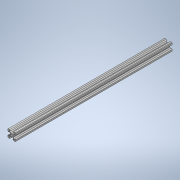
# Autodesk Inventor part: 2020
Saved by Autodesk Inventor 2020 (Build 240168000, 168)
## iProperties
Created: 2021-03-19
Part Number: 2020
Material: Aluminum 6061
Document SubType Name: Modeling
Designer: AOB
Mass: 180.098 g
Surface Area: 658.384 cm^2
Volume: 66.7031 cm^3
Density: 2.7 g/cm^3
Appearance: Anodized - Light Gray
Author: AOB
Autodesk Inventor part; units mm, degrees
ref_plane "YZ Plane" through (0, 0, 0) normal (1, 0, 0) x (0, 1, 0)
ref_plane "XZ Plane" through (0, 0, 0) normal (0, 1, 0) x (-1, 0, 0)
ref_plane "XY Plane" through (0, 0, 0) normal (0, 0, 1) x (1, 0, 0)
sketch "Sketch1" plane through (0, 0, 0) normal (0, 0, 1) x (1, 0, 0)
  line L0 (1, 7) -> (1, 7)
  line L1 (-1, 5) -> (-1, 1)
  arc A0 (-1, 1) -> (0, 0) centre (0, 1) ccw
  line L2 (0, 0) -> (4, 0)
  line L3 (6, 2) -> (6, 2)
  line L4 (6, 2) -> (3, 2)
  line L5 (3, 2) -> (3, 2.9393)
  line L6 (3, 2.9393) -> (6.0607, 6)
  line L7 (6.0607, 6) -> (11.9393, 6)
  line L8 (11.9393, 6) -> (15, 2.9393)
  line L9 (15, 2.9393) -> (15, 2)
  line L10 (15, 2) -> (12, 2)
  line L11 (12, 2) -> (12, 2)
  line L12 (14, 0) -> (18, 0)
  arc A1 (18, 0) -> (19, 1) centre (18, 1) ccw
  line L13 (19, 1) -> (19, 5)
  line L14 (17, 7) -> (17, 7)
  line L15 (17, 7) -> (17, 4)
  line L16 (17, 4) -> (16.0607, 4)
  line L17 (16.0607, 4) -> (13, 7.0607)
  line L18 (13, 7.0607) -> (13, 9.4804)
  line L19 (13, 7.0607) -> (13, 12.9393)
  line L20 (13, 12.9393) -> (16.0607, 16)
  line L21 (16.0607, 16) -> (17, 16)
  line L22 (17, 16) -> (17, 13)
  line L23 (17, 13) -> (17, 13)
  line L24 (19, 15) -> (19, 19)
  arc A2 (19, 19) -> (18, 20) centre (18, 19) ccw
  line L25 (18, 20) -> (14, 20)
  line L26 (12, 18) -> (12, 18)
  line L27 (12, 18) -> (15, 18)
  line L28 (15, 18) -> (15, 17.0607)
  line L29 (15, 17.0607) -> (11.9393, 14)
  line L30 (11.9393, 14) -> (9.5196, 14)
  line L31 (11.9393, 14) -> (6.0607, 14)
  line L32 (6.0607, 14) -> (3, 17.0607)
  line L33 (3, 17.0607) -> (3, 18)
  line L34 (3, 18) -> (6, 18)
  line L35 (6, 18) -> (6, 18)
  line L36 (4, 20) -> (0, 20)
  arc A3 (0, 20) -> (-1, 19) centre (0, 19) ccw
  line L37 (-1, 19) -> (-1, 15)
  line L38 (1, 13) -> (1, 13)
  line L39 (1, 13) -> (1, 16)
  line L40 (1, 16) -> (1.9393, 16)
  line L41 (1.9393, 16) -> (5, 12.9393)
  line L42 (5, 12.9393) -> (5, 7.0607)
  line L43 (5, 9.4804) -> (5, 7.0607)
  line L44 (5, 7.0607) -> (1.9393, 4)
  line L45 (1.9393, 4) -> (1, 4)
  line L46 (1, 4) -> (1, 7)
  circle A4 centre (9, 10) radius 2.1
  line L47 (6, 18) -> (4, 20)
  line L48 (12, 18) -> (14, 20)
  line L49 (1, 13) -> (-1, 15)
  line L50 (1, 7) -> (-1, 5)
  line L51 (19, 15) -> (17, 13)
  line L52 (19, 5) -> (17, 7)
  line L53 (6, 2) -> (4, 0)
  line L54 (12, 2) -> (14, 0)
  point P0 (-1, 7)
  point P1 (6, 0)
  point P2 (12, 0)
  point P3 (19, 7)
  point P4 (19, 13)
  point P5 (12, 20)
  point P6 (6, 20)
  point P7 (-1, 13)
  dimension "d0" = 2
  dimension "d1" = 2
  dimension "d2" = 2
  dimension "d3" = 2
  dimension "d4" = 2
  dimension "d5" = 2
  dimension "d6" = 2
  dimension "d7" = 2
  dimension "d8" = 2
  dimension "d9" = 2
  dimension "d10" = 2
  dimension "d11" = 2
  dimension "d12" = 2
  dimension "d13" = 2
  dimension "d14" = 2
  dimension "d15" = 2
  constraints: 110 end point, 16 point on line, 8 point on circle, 5 centre point
  measures "d0" distance of L35.end point (6, 20)
  measures "d1" distance of L36.start point (6, 20)
  measures "d2" distance of L26.start point (12, 20)
  measures "d3" distance of L25.end point (12, 20)
  measures "d4" distance of L38.start point (-1, 13)
  measures "d5" distance of L37.end point (-1, 13)
  measures "d6" distance of L0.end point (-1, 7)
  measures "d7" distance of L1.start point (-1, 7)
  measures "d8" distance of L24.start point (19, 13)
  measures "d9" distance of L23.end point (19, 13)
  measures "d10" distance of L13.end point (19, 7)
  measures "d11" distance of L14.start point (19, 7)
  measures "d12" distance of L3.start point (6, 0)
  measures "d13" distance of L2.end point (6, 0)
  measures "d14" distance of L11.end point (12, 0)
  measures "d15" distance of L12.start point (12, 0)
extrude "Extrusion1" add sketch "Sketch1" along normal blind 400
equation "\"d1\" = d0"
equation "\"d2\" = d0"
equation "\"d3\" = d2"
equation "\"d4\" = d0"
equation "\"d5\" = d4"
equation "\"d6\" = d0"
equation "\"d7\" = d6"
equation "\"d8\" = d0"
equation "\"d9\" = d8"
equation "\"d10\" = d0"
equation "\"d11\" = d10"
equation "\"d12\" = d0"
equation "\"d13\" = d12"
equation "\"d14\" = d0"
equation "\"d15\" = d14"
body "Solid1"
